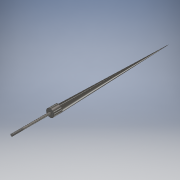
# Autodesk Inventor part: Blade
Saved by Autodesk Inventor 2017 (Build 210142000, 142)
## iProperties
Created: 2019-06-22
Part Number: Blade
Material: Steel
Document SubType Name: Modeling
Designer: Ole Simmering
Density: 7.85 g/cm^3
Appearance: Steel - Polished
Author: Ole Simmering
Autodesk Inventor part; units mm, degrees
ref_plane "YZ Plane" through (0, 0, 0) normal (1, 0, 0) x (0, 1, 0)
ref_plane "XZ Plane" through (0, 0, 0) normal (0, 1, 0) x (-1, 0, 0)
ref_plane "XY Plane" through (0, 0, 0) normal (0, 0, 1) x (1, 0, 0)
sketch "Sketch1" plane through (0, 0, 0) normal (0, 1, 0) x (-1, 0, 0)
  circle A0 centre (0, 0) radius 2
  constraints: 1 centre point, 1 coincident
extrude "Extrusion1" add sketch "Sketch1" along normal blind 70
sketch "Sketch3" plane through (0, 70, 0) normal (0, 1, 0) x (1, 0, 0)
  circle A0 centre (0, 0) radius 7
  dimension "d18" = 14
  constraints: 1 centre point, 1 coincident
  measures "d18" diameter of A0
extrude "Extrusion2" add sketch "Sketch3" along normal blind 15
sketch "Sketch4" plane through (0, 85, 0) normal (0, 1, 0) x (1, 0, 0)
  line L0 (-42, 0) -> (0, 0) construction
  line L1 (0, 0) -> (43.0694, 0) construction
  circle A0 centre (0, 0) radius 2 construction
  line L2 (0, 0) -> (-13.8564, 24) construction
  line L3 (0, 0) -> (27.7128, 0) construction
  line L4 (0, 0) -> (21.6109, -37.4311) construction
  line L5 (0, 0) -> (-14.4338, -25) construction
  line L6 (0, 0) -> (28.8675, 0) construction
  line L7 (0, 0) -> (22.7278, 39.3656) construction
  circle A1 centre (0, 0) radius 7 construction
  arc A2 (3.5, -6.0622) -> (-7, 0) centre (-13.8769, -24.0356) ccw
  arc A3 (3.5, 6.0622) -> (3.5, -6.0622) centre (27.7539, 0) ccw
  arc A4 (-7, 0) -> (3.5, 6.0622) centre (-13.8769, 24.0356) ccw
  circle A5 centre (0, 0) radius 7 construction
  dimension "d21" = 120
  dimension "d22" = 120
  dimension "d27" = 25
  dimension "d28" = 25
  dimension "d29" = 25
  constraints: 17 end point, 8 point on circle, 3 centre point, 3 collinear, 3 horizontal, 3 point on line, 2 equal length, 2 other
  measures "d21" angle of L3 L2
  measures "d22" angle of L5 L6
  measures "d27" radius of A2
  measures "d28" radius of A3
  measures "d29" radius of A4
ref_plane "Work Plane1" through (0, 285, 0) normal (0, 1, 0) x (1, 0, 0)
sketch "Sketch5" plane through (0, 285, 0) normal (0, 1, 0) x (1, 0, 0)
  circle A0 centre (0, 0) radius 0.0063
  dimension "d31" = 0.0125
  constraints: 1 centre point, 1 coincident
  measures "d31" diameter of A0
loft "Loft1" add profiles "Sketch4", "Sketch5"
thread "Thread1" size "M4x0.7" class "6g" standard "ANSI Metric M Profile" length 20
equation "\"d28\" = d27"
equation "\"d29\" = d27"
body "Solid1"
